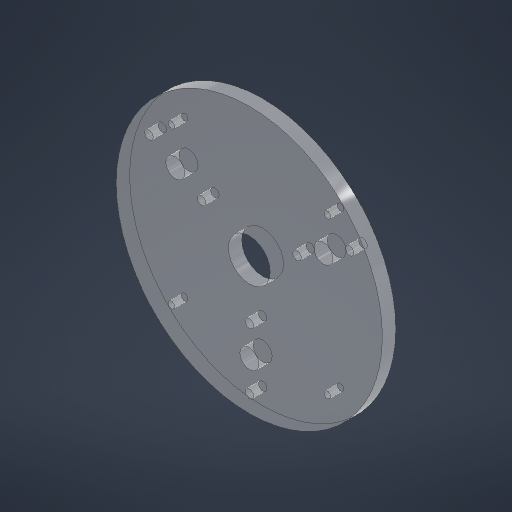
# Autodesk Inventor part: SupBase
Saved by Autodesk Inventor 2025.2 (Build 292293000, 293)
## iProperties
Created: 2025-04-27
Part Number: SupBase
Material: Generic
Document SubType Name: Modeling
Designer: Tiago
Density: 1 g/cm^3
Appearance: Polycarbonate - Clear
Author: Tiago
Autodesk Inventor part; units mm, degrees
ref_plane "YZ Plane" through (0, 0, 0) normal (1, 0, 0) x (0, 1, 0)
ref_plane "XZ Plane" through (0, 0, 0) normal (0, 1, 0) x (-1, 0, 0)
ref_plane "XY Plane" through (0, 0, 0) normal (0, 0, 1) x (1, 0, 0)
sketch "Sketch1" plane through (0, 0, 0) normal (0, 0, 1) x (1, 0, 0)
  circle A0 centre (0, 0) radius 70
  line L0 (-41, 0) -> (41, 0) construction
  line L1 (0, -41) -> (0, 41) construction
  line L2 (0, 41) -> (41, 41) construction
  line L3 (41, 41) -> (41, 0) construction
  circle A1 centre (41, 41) radius 1.75
  circle A2 centre (41, -41) radius 1.75
  circle A3 centre (-41, 41) radius 1.75
  circle A4 centre (-41, -41) radius 1.75
  circle A5 centre (41, 41) radius 5 construction
  circle A6 centre (41, -41) radius 5 construction
  circle A7 centre (-41, -41) radius 5 construction
  circle A8 centre (-41, 41) radius 5 construction
  line L4 (0, 0) -> (0, -45) construction
  circle A9 centre (0, 0) radius 45 construction
  circle A10 centre (0, 0) radius 11
  circle A11 centre (0, -45) radius 5
  line L5 (0, -61) -> (0, -29) construction
  circle A12 centre (0, -61) radius 2.25
  circle A13 centre (0, -29) radius 2.25
  circle A14 centre (52.8275, 30.5) radius 2.25
  line L6 (52.8275, 30.5) -> (25.1147, 14.5) construction
  circle A15 centre (38.9711, 22.5) radius 5
  circle A16 centre (25.1147, 14.5) radius 2.25
  circle A17 centre (-52.8275, 30.5) radius 2.25
  line L7 (-52.8275, 30.5) -> (-25.1147, 14.5) construction
  circle A18 centre (-38.9711, 22.5) radius 5
  circle A19 centre (-25.1147, 14.5) radius 2.25
  point P0 (38.9711, 22.5)
  dimension "d0" = 140
  dimension "L_furos" = 82
  dimension "d2" = 82
  dimension "d3" = 3.5
  dimension "d4" = 10
  dimension "d5" = 45
  dimension "d24" = 360
  dimension "d49" = 22
  dimension "d52" = 10
  dimension "d54" = 32
  dimension "d55" = 4.5
  dimension "d56" = 4.5
  dimension "d59" = 360
  constraints: 19 centre point, 16 end point, 12 coincident, 6 symmetric about line, 3 midpoint, 2 horizontal, 2 vertical, 1 perpendicular, 1 point on line, 41 other
  measures "d0" diameter of A0
  measures "L_furos" distance of L0.start L0.end
  measures "d2" distance of L1.start L1.end
  measures "d3" diameter of A1
  measures "d4" diameter of A5
  measures "d5" distance of L4.start L4.end
  measures "d49" diameter of A10
  measures "d52" diameter of A11
  measures "d54" distance of L5.start L5.end
  measures "d55" diameter of A12
  measures "d56" diameter of A13
extrude "Extrusion1" add sketch "Sketch1" along normal blind 7
equation "\"d2\" = L_furos"
equation "\"d21\" = 5.5"
equation "\"d39\" = 5.5"
body "Solid1"
